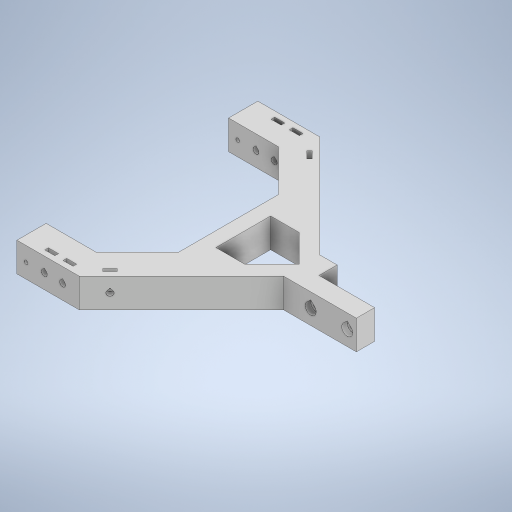
# Autodesk Inventor part: middle_Y
Saved by Autodesk Inventor 2023.1 (Build 271208000, 208)
## iProperties
Created: 2023-11-20
Part Number: middle_Y
Material: Všeobecné
Document SubType Name: Modeling
Designer: zavrel
Density: 1 g/cm^3
Appearance: Výchozí
Author: zavrel
Autodesk Inventor part; units mm, degrees
ref_plane "YZ Plane" through (0, 0, 0) normal (1, 0, 0) x (0, 1, 0)
ref_plane "XZ Plane" through (0, 0, 0) normal (0, 1, 0) x (-1, 0, 0)
ref_plane "XY Plane" through (0, 0, 0) normal (0, 0, 1) x (1, 0, 0)
sketch "Náčrt1" plane through (0, 0, 0) normal (0, 1, 0) x (-1, 0, 0)
  line L0 (0, 0) -> (0, 10)
  line L1 (0, 10) -> (40, 10)
  line L2 (40, 10) -> (96, 66)
  line L3 (96, 66) -> (130, 66)
  line L4 (130, 66) -> (130, 50)
  line L5 (130, 50) -> (102.6274, 50)
  line L6 (102.6274, 50) -> (80, 27.3726)
  line L7 (80, 27.3726) -> (80, 0)
  line L8 (0, 0) -> (258.3801, 0) construction
  line L9 (0, 0) -> (0, -10)
  line L10 (0, -10) -> (40, -10)
  line L11 (40, -10) -> (96, -66)
  line L12 (96, -66) -> (130, -66)
  line L13 (130, -66) -> (130, -50)
  line L14 (130, -50) -> (102.6274, -50)
  line L15 (102.6274, -50) -> (80, -27.3726)
  line L16 (80, -27.3726) -> (80, 0)
  dimension "d0" = 16
  dimension "d2" = 16
  dimension "d3" = 45
  dimension "d4" = 10
  dimension "d5" = 40
  dimension "d7" = 100
  dimension "d9" = 80
  dimension "d10" = 50
  constraints: 34 end point, 7 symmetric about line, 3 perpendicular, 2 horizontal, 2 parallel, 1 point on line, 1 vertical
  measures "d0" distance of L3.end L4.end
  measures "d2" distance between parallel lines of L6 L2
  measures "d3" angle of L8 L2
  measures "d4" distance between parallel lines of L8 L1
  measures "d5" distance of L9.end L10.end
  measures "d7" distance between parallel lines of L14 L5
  measures "d9" distance between parallel lines of L9 L16
  measures "d10" distance between parallel lines of L16 L13
extrude "Vysunutí1" add sketch "Náčrt1" along normal blind 16
sketch "Náčrt2" plane through (-96, 0, -66) normal (0, 0, -1) x (-1, 0, 0)
  line L0 (0, 0) -> (34, 0) projected
  line L1 (34, 0) -> (34, 16) projected
  line L2 (0, 16) -> (34, 16) projected
  line L3 (0, 0) -> (0, 16) projected
  line L4 (34, 8) -> (0, 8) construction
  circle A0 centre (29, 8) radius 1
  circle A1 centre (19, 8) radius 1.6
  circle A2 centre (9, 8) radius 1.6
  line L5 (19, 8) -> (19, 11.8271) construction
  line L6 (19, 10.2627) -> (20.1314, 9.1314)
  line L7 (19, 10.2627) -> (17.8686, 9.1314)
  line L8 (9, 10.2627) -> (10.1314, 9.1314)
  line L9 (9, 10.2627) -> (7.8686, 9.1314)
  point P0 (-96, 0)
  point P1 (7.8686, 9.1314)
  point P2 (10.1314, 9.1314)
  dimension "d13" = 2
  dimension "d14" = 3.2
  dimension "d15" = 5
  dimension "d16" = 10
  dimension "d17" = 10
  dimension "d22" = 90
  dimension "d23" = 90
  constraints: 12 end point, 4 point on line, 3 centre point, 2 midpoint, 2 point on circle, 2 tangent, 1 equal radius, 1 vertical
  measures "d13" diameter of A0
  measures "d14" diameter of A1
  measures "d15" distance from line of L1 A0.centre
  measures "d16" distance of A0.centre L5.start
  measures "d17" distance of L5.start A2.centre
  measures "d22" angle of L7 L6
  measures "d23" angle of L9 L8
extrude "Vysunutí2" cut sketch "Náčrt2" against normal up to surface (132 mm away) contours A0 | A1 | A1 L7 L6 | A2 | A2 L9 L8
sketch "Náčrt3" plane through (-96, 0, -66) normal (0.7071068, 0, -0.7071068) x (-0.7071068, 0, -0.7071068)
  line L0 (-79.196, 0) -> (0, 0) projected
  line L1 (0, 0) -> (0, 16) projected
  line L2 (-79.196, 16) -> (0, 16) projected
  line L3 (-79.196, 0) -> (-79.196, 16) projected
  line L4 (0, 8) -> (-20.1825, 8) construction
  circle A0 centre (-12, 8) radius 1.6
  line L5 (-12, 8) -> (-12, 19.2417) construction
  line L6 (-12, 10.2627) -> (-10.8686, 9.1314)
  line L7 (-12, 10.2627) -> (-13.1314, 9.1314)
  point P0 (-114.5513, 0)
  dimension "d20" = 3.2
  dimension "d21" = 90
  dimension "d26" = 12
  constraints: 8 end point, 2 point on circle, 2 point on line, 2 tangent, 1 centre point, 1 horizontal, 1 midpoint, 1 vertical
  measures "d20" diameter of A0
  measures "d21" angle of L7 L6
  measures "d26" distance from line of L1 L5.start
extrude "Vysunutí3" cut sketch "Náčrt3" against normal up to surface (16 mm away) contours A0 | A0 L7 L6
sketch "Náčrt4" plane through (-40, 0, 10) normal (0.7071068, 0, 0.7071068) x (0.7071068, 0, -0.7071068)
  line L0 (-79.196, 0) -> (0, 0) projected
  line L1 (0, 0) -> (0, 16) projected
  line L2 (-79.196, 16) -> (0, 16) projected
  line L3 (-79.196, 0) -> (-79.196, 16) projected
  line L4 (-79.196, 8) -> (0, 8) construction
  circle A0 centre (-67.196, 8) radius 1.6
  line L5 (-67.196, 8) -> (-67.196, 16) construction
  line L6 (-67.196, 10.2627) -> (-68.3273, 9.1314)
  line L7 (-67.196, 10.2627) -> (-66.0646, 9.1314)
  point P0 (35.3553, 0)
  dimension "d27" = 3.2
  dimension "d28" = 12
  dimension "d29" = 90
  constraints: 8 end point, 3 point on line, 2 midpoint, 2 point on circle, 2 tangent, 1 centre point, 1 perpendicular
  measures "d27" diameter of A0
  measures "d28" distance from line of L3 L5.start
  measures "d29" angle of L7 L6
extrude "Vysunutí4" cut sketch "Náčrt4" against normal up to surface (16 mm away) contours A0 | A0 L6 L7
sketch "Sketch6" plane through (0, 16, 0) normal (0, 1, 0) x (1, 0, 0)
  line L0 (-130, -66) -> (-96, -66) projected
  line L1 (-96, -66) -> (-40, -10) projected
  line L2 (-96, 66) -> (-130, 66) projected
  line L3 (-40, 10) -> (-96, 66) projected
  line L4 (-117.75, -63) -> (-112.25, -63)
  line L5 (-112.25, -63) -> (-112.25, -61)
  line L6 (-112.25, -61) -> (-117.75, -61)
  line L7 (-117.75, -61) -> (-117.75, -63)
  line L8 (-117.75, -63) -> (-112.25, -61) construction
  line L9 (-112.25, -63) -> (-117.75, -61) construction
  line L10 (-107.75, -63) -> (-102.25, -63)
  line L11 (-102.25, -63) -> (-102.25, -61)
  line L12 (-102.25, -61) -> (-107.75, -61)
  line L13 (-107.75, -61) -> (-107.75, -63)
  line L14 (-107.75, -63) -> (-102.25, -61) construction
  line L15 (-102.25, -63) -> (-107.75, -61) construction
  line L16 (-87.6915, -53.4489) -> (-91.5806, -57.3379)
  line L17 (-91.5806, -57.3379) -> (-92.9948, -55.9237)
  line L18 (-92.9948, -55.9237) -> (-89.1057, -52.0346)
  line L19 (-89.1057, -52.0346) -> (-87.6915, -53.4489)
  line L20 (-87.6915, -53.4489) -> (-92.9948, -55.9237) construction
  line L21 (-91.5806, -57.3379) -> (-89.1057, -52.0346) construction
  line L22 (-130, -50) -> (-130, -66) projected
  line L23 (-96, -66) -> (-99.792, -62.208) construction
  line L24 (-80, 27.3726) -> (-80, -27.3726) projected
  line L25 (-80, 0) -> (-94.3726, 0) construction
  line L26 (-117.75, 63) -> (-112.25, 63)
  line L27 (-112.25, 63) -> (-112.25, 61)
  line L28 (-112.25, 61) -> (-117.75, 61)
  line L29 (-117.75, 61) -> (-117.75, 63)
  line L30 (-117.75, 63) -> (-112.25, 61) construction
  line L31 (-112.25, 63) -> (-117.75, 61) construction
  line L32 (-107.75, 63) -> (-102.25, 63)
  line L33 (-102.25, 63) -> (-102.25, 61)
  line L34 (-102.25, 61) -> (-107.75, 61)
  line L35 (-107.75, 61) -> (-107.75, 63)
  line L36 (-107.75, 63) -> (-102.25, 61) construction
  line L37 (-102.25, 63) -> (-107.75, 61) construction
  line L38 (-87.6915, 53.4489) -> (-91.5806, 57.3379)
  line L39 (-91.5806, 57.3379) -> (-92.9948, 55.9237)
  line L40 (-92.9948, 55.9237) -> (-89.1057, 52.0346)
  line L41 (-89.1057, 52.0346) -> (-87.6915, 53.4489)
  line L42 (-87.6915, 53.4489) -> (-92.9948, 55.9237) construction
  line L43 (-91.5806, 57.3379) -> (-89.1057, 52.0346) construction
  point P0 (0, 0)
  point P1 (-115, -62)
  point P2 (-105, -62)
  point P3 (-90.3431, -54.6863)
  point P4 (-115, 62)
  point P5 (-105, 62)
  point P6 (-90.3431, 54.6863)
  dimension "d53" = 2
  dimension "d54" = 5.5
  dimension "d55" = 15
  dimension "d56" = 10
  dimension "d57" = 12
  dimension "d60" = 3
  dimension "d61" = 3
  constraints: 76 end point, 15 symmetric about line, 9 midpoint, 8 parallel, 4 equal length, 3 horizontal, 3 perpendicular, 2 point on line
  measures "d53" distance of L6.end L4.start
  measures "d54" distance of L5.end L6.end
  measures "d55" distance from line of L22 point (-115, -62)
  measures "d56" distance of point (-105, -62) point (-115, -62)
  measures "d57" distance from line of point (-90.343, -54.686) L23
  measures "d60" distance between parallel lines of L1 L16
  measures "d61" distance between parallel lines of L0 L10
extrude "Extrusion5" cut sketch "Sketch6" against normal blind 11
sketch "Sketch7" plane through (0, 0, -10) normal (0, 0, -1) x (-1, 0, 0)
  line L0 (0, 0) -> (40, 0) projected
  line L1 (40, 0) -> (40, 16) projected
  line L2 (0, 16) -> (40, 16) projected
  line L3 (0, 0) -> (0, 16) projected
  line L4 (0, 8) -> (40, 8) construction
  line L5 (40, 0) -> (40, 16) construction
  circle A0 centre (5, 8) radius 1.6
  circle A1 centre (25, 8) radius 1.6
  line L6 (5, 8) -> (5, 13.898) construction
  line L7 (5, 10.2627) -> (3.8686, 9.1314)
  line L8 (5, 10.2627) -> (6.1314, 9.1314)
  line L9 (25, 10.2627) -> (23.8686, 9.1314)
  line L10 (25, 10.2627) -> (26.1314, 9.1314)
  dimension "d62" = 3.2
  dimension "d63" = 5
  dimension "d64" = 20
  dimension "d65" = 90
  dimension "d66" = 90
  constraints: 12 end point, 3 point on line, 1 centre point, 1 midpoint, 1 vertical, 7 other
  measures "d63" distance from line of L3 L6.start
  measures "d64" distance of A1.centre L6.start
  measures "d65" angle of L8 L7
  measures "d66" angle of L10 L9
extrude "Extrusion6" cut sketch "Sketch7" against normal through all contours A0 | A0 L7 L8 | A1 | A1 L9 L10
sketch "Sketch8" plane through (0, 0, -10) normal (0, 0, -1) x (-1, 0, 0)
  line L0 (23.8686, 9.1314) -> (25, 10.2627) projected
  line L1 (25, 10.2627) -> (26.1314, 9.1314) projected
  arc A0 (23.8686, 9.1314) -> (26.1314, 9.1314) centre (25, 8) ccw projected
  line L2 (3.8686, 9.1314) -> (5, 10.2627) projected
  line L3 (5, 10.2627) -> (6.1314, 9.1314) projected
  arc A1 (3.8686, 9.1314) -> (6.1314, 9.1314) centre (5, 8) ccw projected
  line L4 (0, 0) -> (40, 0) projected
  line L5 (40, 0) -> (40, 16) projected
  line L6 (0, 16) -> (40, 16) projected
  line L7 (0, 0) -> (0, 16) projected
  line L8 (40, 16) -> (0, 16) projected
  line L9 (30.5, 16) -> (30.5, 0)
  line L10 (0, 0) -> (40, 0) projected
  dimension "d69" = 30.5
  constraints: 2 end point, 2 point on line, 1 perpendicular
  measures "d69" distance between parallel lines of L9 L7
extrude "Extrusion7" cut sketch "Sketch8" against normal blind 10 contours L7 L6 L9 L4
sketch "Sketch9" plane through (0, 16, 0) normal (0, 1, 0) x (1, 0, 0)
  line L0 (-80, 27.3726) -> (-80, -27.3726) construction
  line L1 (-80, 0) -> (-30.6313, 0) construction
  line L2 (-72, 0) -> (-72, -15)
  line L3 (-72, -15) -> (-56.3137, -15)
  line L4 (-56.3137, -15) -> (-41.3137, 0)
  line L5 (0, 0) -> (-30.5, 0) projected
  line L6 (-30.5, 0) -> (-30.5, 10) projected
  line L7 (-30.5, 10) -> (-40, 10) projected
  line L8 (-40, 10) -> (-96, 66) projected
  line L9 (-96, 66) -> (-130, 66) projected
  line L10 (-130, 66) -> (-130, 50) projected
  line L11 (-130, 50) -> (-102.6274, 50) projected
  line L12 (-102.6274, 50) -> (-80, 27.3726) projected
  line L13 (-80, 27.3726) -> (-80, -27.3726) projected
  line L14 (-80, -27.3726) -> (-102.6274, -50) projected
  line L15 (-102.6274, -50) -> (-130, -50) projected
  line L16 (-130, -50) -> (-130, -66) projected
  line L17 (-130, -66) -> (-96, -66) projected
  line L18 (-96, -66) -> (-40, -10) projected
  line L19 (-40, -10) -> (0, -10) projected
  line L20 (0, -10) -> (0, 0) projected
  line L21 (-112.25, 63) -> (-112.25, 61) projected
  line L22 (-112.25, 61) -> (-117.75, 61) projected
  line L23 (-117.75, 61) -> (-117.75, 63) projected
  line L24 (-117.75, 63) -> (-112.25, 63) projected
  line L25 (-107.75, -61) -> (-102.25, -61) projected
  line L26 (-102.25, -61) -> (-102.25, -63) projected
  line L27 (-102.25, -63) -> (-107.75, -63) projected
  line L28 (-107.75, -63) -> (-107.75, -61) projected
  line L29 (-117.75, -61) -> (-112.25, -61) projected
  line L30 (-112.25, -61) -> (-112.25, -63) projected
  line L31 (-112.25, -63) -> (-117.75, -63) projected
  line L32 (-117.75, -63) -> (-117.75, -61) projected
  line L33 (-107.75, 61) -> (-107.75, 63) projected
  line L34 (-107.75, 63) -> (-102.25, 63) projected
  line L35 (-102.25, 63) -> (-102.25, 61) projected
  line L36 (-102.25, 61) -> (-107.75, 61) projected
  line L37 (-91.5806, -57.3379) -> (-92.9948, -55.9237) projected
  line L38 (-92.9948, -55.9237) -> (-89.1057, -52.0346) projected
  line L39 (-89.1057, -52.0346) -> (-87.6915, -53.4489) projected
  line L40 (-87.6915, -53.4489) -> (-91.5806, -57.3379) projected
  line L41 (-87.6915, 53.4489) -> (-89.1057, 52.0346) projected
  line L42 (-89.1057, 52.0346) -> (-92.9948, 55.9237) projected
  line L43 (-92.9948, 55.9237) -> (-91.5806, 57.3379) projected
  line L44 (-91.5806, 57.3379) -> (-87.6915, 53.4489) projected
  line L45 (-72, 0) -> (-72, 15)
  line L46 (-72, 15) -> (-56.3137, 15)
  line L47 (-56.3137, 15) -> (-41.3137, 0)
  line L48 (-96, -66) -> (-40, -10) projected
  dimension "d72" = 30
  dimension "d73" = 8
  dimension "d74" = 8
  constraints: 14 end point, 2 point on line, 2 symmetric about line, 1 horizontal, 1 midpoint, 1 parallel, 1 perpendicular, 1 vertical
  measures "d72" distance between parallel lines of L46 L3
  measures "d73" distance between parallel lines of L0 L2
  measures "d74" distance between parallel lines of L18 L4
extrude "Extrusion8" cut sketch "Sketch9" against normal through all contours L45 L46 L47 L4 L3 L2
sketch "Sketch10" plane through (-40, 0, 10) normal (0, 0, 1) x (1, 0, 0)
  line L0 (15, 10.2627) -> (16.1314, 9.1314) projected
  arc A0 (13.8686, 9.1314) -> (16.1314, 9.1314) centre (15, 8) ccw projected
  line L1 (13.8686, 9.1314) -> (15, 10.2627) projected
  line L2 (35, 10.2627) -> (36.1314, 9.1314) projected
  arc A1 (33.8686, 9.1314) -> (36.1314, 9.1314) centre (35, 8) ccw projected
  line L3 (33.8686, 9.1314) -> (35, 10.2627) projected
  line L4 (0, 0) -> (40, 0) projected
  line L5 (40, 0) -> (40, 16) projected
  line L6 (0, 16) -> (40, 16) projected
  line L7 (0, 0) -> (0, 16) projected
  arc A2 (13.8686, 9.1314) -> (16.1314, 9.1314) centre (15, 8) ccw projected
  circle A3 centre (15, 8) radius 3
  circle A4 centre (35, 8) radius 3
  line L8 (15, 12.2426) -> (12.8787, 10.1213)
  line L9 (15, 12.2426) -> (17.1213, 10.1213)
  line L10 (35, 12.2426) -> (32.8787, 10.1213)
  line L11 (35, 12.2426) -> (37.1213, 10.1213)
  dimension "d77" = 6
  dimension "d78" = 6
  dimension "d79" = 90
  dimension "d80" = 90
  constraints: 8 end point, 2 centre point, 2 coincident, 2 point on circle, 2 tangent, 1 parallel
  measures "d77" diameter of A3
  measures "d78" diameter of A4
  measures "d79" angle of L9 L8
  measures "d80" angle of L11 L10
extrude "Extrusion9" cut sketch "Sketch10" against normal blind 3 contours A3 | A3 L8 L9 | A4 | A4 L10 L11
